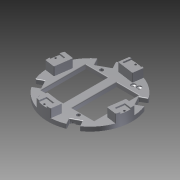
# Autodesk Inventor part: flush floor outlet cover part 1
Saved by Autodesk Inventor 2012 (Build 160160000, 160)
## iProperties
Created: 2012-03-08
Part Number: flush floor outlet cover part 1
Material: Default
Document SubType Name: Modeling
Designer: 21842
Density: 1 g/cm^3
Author: 21842
Autodesk Inventor part; units mm, degrees
sketch "Sketch2" plane through (0, 0, 0) normal (0, 1, 0) x (-1, 0, 0)
  circle A0 centre (0, 0) radius 63
  dimension "d0" = 126
  constraints: 1 centre point, 1 coincident
  measures "d0" diameter of A0
extrude "Extrusion1" add sketch "Sketch2" along normal blind 6.35
sketch "Sketch3" plane through (0, 6.35, 0) normal (0, 1, 0) x (1, 0, 0)
  circle A0 centre (0, 0) radius 63 projected
  line L0 (39.8375, 33.4) -> (39.8375, -33.4)
  line L1 (39.8375, 33.4) -> (6.5, 33.4)
  line L2 (6.5, 33.4) -> (6.5, -33.4)
  line L3 (6.5, -33.4) -> (39.8375, -33.4)
  line L4 (-39.8375, 33.3313) -> (-39.8375, -33.4687)
  line L5 (-39.8375, 33.3313) -> (-6.5, 33.3313)
  line L6 (-6.5, 33.3313) -> (-6.5, -33.4687)
  line L7 (-6.5, -33.4687) -> (-39.8375, -33.4687)
  point P0 (39.8375, 0)
  point P1 (6.5, 0)
  point P2 (-36.1156, 0)
  point P3 (-2.7781, 0)
  dimension "d4" = 33.3375
  dimension "d5" = 66.8
  dimension "d6" = 6.5
  dimension "d180" = 66.8
  dimension "d181" = 66.8
  dimension "d182" = 33.3375
  dimension "d218" = 6.5
  constraints: 12 end point, 2 horizontal, 2 midpoint, 2 parallel, 2 perpendicular, 1 horizontal alignment, 6 other
  measures "d4" distance of L0.start L1.end
  measures "d5" distance of L0.start L0.end
  measures "d6" distance from line of L2 A0.centre
  measures "d180" distance of L5.start L7.end
  measures "d181" distance of L5.end L7.start
  measures "d182" distance of L5.start L5.end
extrude "Extrusion2" cut sketch "Sketch3" against normal through all contours L0 L3 L2 L1 | L5 L6 L7 L4
ref_plane "Work Plane5" through (0, 6.35, 0) normal (0, 1, 0) x (1, 0, 0)
sketch "Sketch21" plane through (0, 6.35, 0) normal (0, 1, 0) x (1, 0, 0)
  line L0 (-44.4846, 19.0767) -> (-48.0196, -6.0761)
  line L1 (-44.4846, 19.0767) -> (-59.3386, 21.1643)
  line L2 (-48.0196, -6.0761) -> (-62.8736, -3.9885)
  line L3 (-19.0767, -44.4846) -> (6.0761, -48.0196)
  line L4 (-19.0767, -44.4846) -> (-21.1643, -59.3386)
  line L5 (6.0761, -48.0196) -> (3.9885, -62.8736)
  line L6 (44.4846, -19.0767) -> (48.0196, 6.0761)
  line L7 (44.4846, -19.0767) -> (59.3386, -21.1643)
  line L8 (48.0196, 6.0761) -> (62.8736, 3.9885)
  line L9 (19.0767, 44.4846) -> (-6.0761, 48.0196)
  line L10 (19.0767, 44.4846) -> (21.1643, 59.3386)
  line L11 (-6.0761, 48.0196) -> (-3.9885, 62.8736)
  arc A0 (-59.3386, 21.1643) -> (-62.8736, -3.9885) centre (0, 0) ccw
  arc A1 (-21.1643, -59.3386) -> (3.9885, -62.8736) centre (0, 0) ccw
  arc A2 (59.3386, -21.1643) -> (62.8736, 3.9885) centre (0, 0) ccw
  arc A3 (21.1643, 59.3386) -> (-3.9885, 62.8736) centre (0, 0) ccw
  point P0 (-46.2521, 6.5003)
  point P1 (-6.5003, -46.2521)
  point P2 (46.2521, -6.5003)
  point P3 (6.5003, 46.2521)
  dimension "d149" = 25.4
  dimension "d150" = 15
  dimension "d153" = 360
  constraints: 24 end point, 8 point on circle, 4 centre point, 1 coincident, 1 midpoint, 1 perpendicular, 33 other
  measures "d149" distance of L0.start L0.end
  measures "d150" distance of L0.start L1.end
extrude "Extrusion14" add sketch "Sketch21" along normal blind 12.7
ref_plane "Work Plane4" through (0, 6.35, 0) normal (0, 1, 0) x (1, 0, 0)
sketch "Sketch7" plane through (0, 6.35, 0) normal (0, 1, 0) x (1, 0, 0)
  line L0 (-62.213, -25.5347) -> (-49.2176, -18.5043)
  line L1 (-62.213, -25.5347) -> (-55.4146, -38.1011)
  line L2 (-55.4146, -38.1011) -> (-42.4193, -31.0707)
  line L3 (-49.2176, -18.5043) -> (-42.4193, -31.0707)
  circle A0 centre (0, 0) radius 63 projected
  line L4 (-32.6825, 39.3958) -> (-15.0917, 48.9123)
  line L5 (-32.6825, 39.3958) -> (-40.9604, 54.6971)
  line L6 (-15.0917, 48.9123) -> (-23.4443, 64.3518)
  line L7 (-40.9604, 54.6971) -> (-23.4443, 64.3518)
  line L8 (25.5347, -62.213) -> (18.5043, -49.2176)
  line L9 (25.5347, -62.213) -> (38.1011, -55.4146)
  line L10 (38.1011, -55.4146) -> (31.0707, -42.4193)
  line L11 (18.5043, -49.2176) -> (31.0707, -42.4193)
  line L12 (62.213, 25.5347) -> (49.2176, 18.5043)
  line L13 (62.213, 25.5347) -> (55.4146, 38.1011)
  line L14 (55.4146, 38.1011) -> (42.4193, 31.0707)
  line L15 (49.2176, 18.5043) -> (42.4193, 31.0707)
  point P0 (-51.6544, -36.0669)
  point P1 (-58.4528, -23.5005)
  point P2 (-38.3924, 49.9502)
  point P3 (-20.8016, 59.4668)
  point P4 (36.0669, -51.6544)
  point P5 (23.5005, -58.4528)
  point P6 (51.6544, 36.0669)
  point P7 (58.4528, 23.5005)
  dimension "d194" = 10.5
  dimension "d195" = 10.5
  dimension "d201" = 20
  dimension "d202" = 12
  dimension "d203" = 12
  dimension "d207" = 270
  constraints: 32 end point, 8 point on line, 4 perpendicular, 4 point on circle, 2 parallel, 21 other
  measures "d194" distance from line of L3 A0.end
  measures "d195" distance from line of L3 A0.start
  measures "d201" distance of L4.start L4.end
  measures "d202" distance from line of L4 point (-38.392, 49.95)
  measures "d203" distance from line of L4 point (-20.802, 59.467)
ref_plane "Work Plane9" through (-40.7136, 31.75, 31.8089) normal (0, -1, 0) x (0.6959411, 0, 0.7180989)
sketch "Sketch23" plane through (0, 19.05, 0) normal (0, 1, 0) x (1, 0, 0)
  line L0 (-52.9864, 0.6304) -> (-51.1075, 13.999)
  line L1 (-51.1075, 13.999) -> (-61.0102, 15.3908)
  line L2 (-52.9864, 0.6304) -> (-62.8891, 2.0221)
  line L3 (-2.41, 51.1124) -> (16.4051, 48.4681)
  line L4 (-2.41, 51.1124) -> (-0.7399, 62.9957)
  line L5 (16.4051, 48.4681) -> (18.0752, 60.3514)
  line L6 (-0.6304, -52.9864) -> (-13.999, -51.1075)
  line L7 (-13.999, -51.1075) -> (-15.3908, -61.0102)
  line L8 (-0.6304, -52.9864) -> (-2.0221, -62.8891)
  line L9 (52.9864, -0.6304) -> (51.1075, -13.999)
  line L10 (51.1075, -13.999) -> (61.0102, -15.3908)
  line L11 (52.9864, -0.6304) -> (62.8891, -2.0221)
  arc A0 (18.0752, 60.3514) -> (-0.7399, 62.9957) centre (0, 0) ccw
  arc A1 (61.0102, -15.3908) -> (62.8891, -2.0221) centre (0, 0) ccw
  arc A2 (-61.0102, 15.3908) -> (-62.8891, 2.0221) centre (0, 0) ccw
  arc A3 (-15.3908, -61.0102) -> (-2.0221, -62.8891) centre (0, 0) ccw
  point P0 (-44.4846, 19.0767)
  point P1 (0, 0)
  point P2 (-19.0767, -44.4846)
  point P3 (44.4846, -19.0767)
  dimension "d166" = 13.5
  dimension "d167" = 10
  dimension "d168" = 10
  dimension "d169" = 19
  dimension "d170" = 12
  dimension "d171" = 12
  dimension "d174" = 270
  constraints: 24 end point, 8 point on circle, 4 centre point, 2 parallel, 2 perpendicular, 1 coincident, 17 other
  measures "d166" distance of L0.start L0.end
  measures "d167" distance of L0.end L1.end
  measures "d168" distance of L0.start L2.end
  measures "d169" distance of L3.start L3.end
  measures "d170" distance of L3.start L4.end
  measures "d171" distance of L3.end L5.end
extrude "Extrusion15" cut sketch "Sketch23" against normal blind 2.25
extrude "Extrusion16" cut sketch "Sketch7" against normal through all contours L0 A0 L2 L1 | L0 L3 L2 A0 | L5 L7 L6 A0 | A0 L6 L4 L5 | L8 L11 L10 A0 | A0 L10 L9 L8 | L14 L13 L12 A0 | A0 L12 L15 L14
sketch "Sketch24" plane through (-52.9864, 16.8, -0.6304) normal (-0.9902681, 0, -0.1391731) x (-0.1391731, 0, 0.9902681)
  line L0 (0, 0) -> (-13.5, 0) projected
  line L1 (0, 2.25) -> (0, 0) projected
  line L2 (-13.5, 2.25) -> (0, 2.25) projected
  line L3 (-13.5, 2.25) -> (-13.5, 0) projected
  point P0 (-6.75, -16.8)
extrude "Extrusion17" cut sketch "Sketch24" along normal blind 100
sketch "Sketch25" plane through (52.9864, 16.8, 0.6304) normal (0.9902681, 0, 0.1391731) x (0.1391731, 0, -0.9902681)
  line L0 (0, 0) -> (-13.5, 0) projected
  line L1 (0, 2.25) -> (0, 0) projected
  line L2 (-13.5, 2.25) -> (0, 2.25) projected
  line L3 (-13.5, 2.25) -> (-13.5, 0) projected
  point P0 (-6.75, -16.8)
extrude "Extrusion18" cut sketch "Sketch25" along normal blind 100
sketch "Sketch26" plane through (-0.6304, 16.8, 52.9864) normal (-0.1391731, 0, 0.9902681) x (0.9902681, 0, 0.1391731)
  line L0 (0, 0) -> (-13.5, 0) projected
  line L1 (0, 2.25) -> (0, 0) projected
  line L2 (-13.5, 2.25) -> (0, 2.25) projected
  line L3 (-13.5, 2.25) -> (-13.5, 0) projected
  point P0 (-6.75, -16.8)
extrude "Extrusion19" cut sketch "Sketch26" along normal blind 100
sketch "Sketch27" plane through (0, 6.35, 0) normal (0, 1, 0) x (1, 0, 0)
  arc A0 (4.1306, -61.8622) -> (58.3273, -21.0222) centre (0, 0) ccw projected
  circle A1 centre (-30.3996, -43.4151) radius 1.6
  circle A2 centre (30.3996, 43.4151) radius 1.6
  point P0 (36.4083, -50.184)
  dimension "d220" = 3.2
  dimension "d223" = 360
  constraints: 2 centre point, 5 other
  measures "d220" diameter of A1
extrude "Extrusion20" cut sketch "Sketch27" against normal through all
sketch "Sketch30" plane through (0, 6.35, 0) normal (0, 1, 0) x (1, 0, 0)
  circle A0 centre (23.1688, 41.9) radius 1.6
  circle A1 centre (-23.1688, -41.9) radius 1.6
  dimension "d235" = 3.2
  constraints: 2 centre point
  measures "d235" diameter of A0
extrude "Extrusion22" cut sketch "Sketch30" against normal through all
ref_plane "Work Plane10" through (62.9672, 16.8, 2.0331) normal (0, 1, 0) x (1, 0, 0)
sketch "Sketch31" plane through (62.9672, 16.8, 2.0331) normal (0, 1, 0) x (1, 0, 0)
  arc A0 (-1.8788, -13.3686) -> (0, 0) centre (-62.9672, 2.0331) ccw projected
  line L0 (-11.8596, -11.9659) -> (-9.9808, 1.4027) projected
  line L1 (-0.5803, -6.7348) -> (-2.9569, -6.4008)
  circle A1 centre (-2.9569, -6.4008) radius 1.6
  circle A2 centre (-54.5333, 62.0434) radius 1.6
  circle A3 centre (-122.9774, 10.467) radius 1.6
  circle A4 centre (-71.4011, -57.9771) radius 1.6
  dimension "d238" = 2.4
  dimension "d239" = 3.2
  dimension "d242" = 360
  constraints: 4 centre point, 2 end point, 1 coincident, 1 point on circle, 9 other
  measures "d238" distance of L1.start L1.end
  measures "d239" diameter of A1
extrude "Extrusion23" cut sketch "Sketch31" against normal through all
sketch "Sketch43" plane through (0, 0, 0) normal (0, -1, 0) x (1, 0, 0)
  circle A0 centre (21.0193, -37.8626) radius 2.5
  circle A1 centre (-20.5794, 37.9797) radius 2.5
  circle A2 centre (-23.1687, 49.2187) radius 3.5
  circle A3 centre (-23.1688, -49.2187) radius 3.5
  circle A4 centre (23.1687, -49.2187) radius 3.5
  arc A5 (62.5878, 7.1951) -> (9.9932, 62.2024) centre (0, 0) ccw
  arc A6 (-10.0069, 62.2002) -> (-62.596, 7.1235) centre (0, 0) ccw
  arc A7 (-62.5914, -7.164) -> (-7.0793, -62.601) centre (0, 0) ccw
  arc A8 (7.2082, -62.5863) -> (62.5995, -7.0924) centre (0, 0) ccw
  circle A9 centre (20.5794, 37.9797) radius 2.75
  circle A10 centre (30.4322, -43.4151) radius 1.6
  circle A11 centre (-30.3669, 43.4151) radius 1.6
  circle A12 centre (23.2014, -41.9) radius 1.6
  circle A13 centre (-23.1361, 41.9) radius 1.6
  circle A14 centre (23.1687, 49.2187) radius 3.5
  circle A15 centre (-20.5794, -37.9797) radius 2.75
  dimension "d266" = 5.5
  dimension "d267" = 5.5
  constraints: 16 centre point, 8 point on circle
  measures "d266" diameter of A9
  measures "d267" diameter of A15
extrude "Extrusion30" cut sketch "Sketch43" against normal blind 2.5 contours A2 | A3 | A4 | A14
extrude "Extrusion31" cut sketch "Sketch43" against normal through all contours A9 | A15
hole "Hole1" at (30.3996, 6.35, -43.4151) direction (0, -1, 0) diameter 7 depth 1.5 tip angle 118
hole "Hole2" at (-30.3996, 6.35, 43.4151) direction (0, -1, 0) diameter 7 depth 1.5 tip angle 118
hole "Hole3" at (23.1688, 6.35, -41.9) direction (0, -1, 0) diameter 7 depth 1.5 tip angle 118
hole "Hole4" at (-23.1688, 6.35, 41.9) direction (0, -1, 0) diameter 7 depth 1.5 tip angle 118
fillet "Fillet15" radius 1 44 edges at (3.9885, 12.7, 62.8736) (6.0761, 12.7, 48.0196) (-21.1643, 12.7, 59.3386) (-19.0767, 12.7, 44.4846) (59.3386, 12.7, 21.1643) (44.4846, 12.7, 19.0767) (62.8736, 12.7, -3.9885) (48.0196, 12.7, -6.0761) (19.0767, 12.7, -44.4846) (-6.0761, 12.7, -48.0196) (21.1643, 12.7, -59.3386) (-3.9885, 12.7, -62.8736) (-59.3386, 12.7, -21.1643) (-44.4846, 12.7, -19.0767) (-48.0196, 12.7, 6.0761) (-62.8736, 12.7, 3.9885) (6.5, 6.35, 0) (23.1688, 6.35, -33.4) (39.8375, 6.35, 0) (23.1688, 6.35, 33.4) (-6.5, 6.35, 0.0687) (-23.1687, 6.35, -33.3313) (-39.8375, 6.35, 0.0687) (-23.1688, 6.35, 33.4687) (-35.5374, 6.35, -44.673) (-23.8871, 6.35, -44.154) (-17.9466, 6.35, -54.1895) (-53.8352, 6.35, 21.0024) (-45.8184, 6.35, 24.7875) (-47.0368, 6.35, 33.5688) (47.0368, 6.35, -33.5688) (33.5688, 6.35, 47.0368) (24.7875, 6.35, 45.8184) (21.0024, 6.35, 53.8352) (45.8184, 6.35, -24.7875) (53.8352, 6.35, -21.0024) (23.5005, 3.175, 58.4528) (36.0669, 3.175, 51.6544) (51.6544, 3.175, -36.0669) (58.4528, 3.175, -23.5005) (-58.4528, 3.175, 23.5005) (-51.6544, 3.175, 36.0669) (-20.8016, 3.175, -59.4668) (-38.3924, 3.175, -49.9502)
fillet "Fillet16" radius 1 16 edges at (18.1073, 6.0571, 49.0994) (18.5043, 2.675, 49.2176) (31.189, 6.0571, 42.0223) (31.0707, 2.675, 42.4193) (42.0223, 6.0571, -31.189) (42.4193, 2.675, -31.0707) (49.0994, 6.0571, -18.1073) (49.2176, 2.675, -18.5043) (-32.6825, 2.675, -39.3958) (-32.8007, 6.0571, -38.9988) (-14.6947, 6.0571, -48.794) (-15.0917, 2.675, -48.9123) (-49.0994, 6.0571, 18.1073) (-49.2176, 2.675, 18.5043) (-42.4193, 2.675, 31.0707) (-42.0223, 6.0571, 31.189)
body "Solid1"
